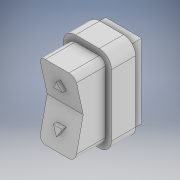
# Autodesk Inventor part: IPC dumb rocker switch
Saved by Autodesk Inventor 2022 (Build 260153000, 153)
## iProperties
Created: 2022-01-05
Part Number: IPC dumb rocker switch
Material: Generic
Document SubType Name: Modeling
Designer: solor
Density: 1 g/cm^3
Appearance: Default
Author: solor
Autodesk Inventor part; units mm, degrees
ref_plane "YZ Plane" through (0, 0, 0) normal (1, 0, 0) x (0, 1, 0)
ref_plane "XZ Plane" through (0, 0, 0) normal (0, 1, 0) x (-1, 0, 0)
ref_plane "XY Plane" through (0, 0, 0) normal (0, 0, 1) x (1, 0, 0)
sketch "Sketch1" plane through (0, 0, 0) normal (0, 0, 1) x (1, 0, 0)
  line L0 (7.88, 0) -> (2, 0)
  arc A0 (7.88, 0) -> (9.88, 2) centre (7.88, 2) ccw
  line L1 (9.88, 17.34) -> (9.88, 2)
  arc A1 (9.88, 17.34) -> (7.88, 19.34) centre (7.88, 17.34) ccw
  line L2 (2, 19.34) -> (7.88, 19.34)
  arc A2 (2, 19.34) -> (0, 17.34) centre (2, 17.34) ccw
  line L3 (0, 2) -> (0, 17.34)
  arc A3 (0, 2) -> (2, 0) centre (2, 2) ccw
  line L4 (0.47, 17.34) -> (0.47, 2)
  arc A4 (0.47, 2) -> (2, 0.47) centre (2, 2) ccw
  line L5 (2, 0.47) -> (7.88, 0.47)
  arc A5 (7.88, 0.47) -> (9.41, 2) centre (7.88, 2) ccw
  line L6 (9.41, 2) -> (9.41, 17.34)
  arc A6 (9.41, 17.34) -> (7.88, 18.87) centre (7.88, 17.34) ccw
  line L7 (7.88, 18.87) -> (2, 18.87)
  arc A7 (2, 18.87) -> (0.47, 17.34) centre (2, 17.34) ccw
  point P0 (0, 0)
  point P1 (0, 0)
  point P2 (0, 0)
  dimension "d0" = 0.47
  constraints: 16 end point, 16 point on circle, 8 centre point, 1 point on line, 7 other
  measures "d0" distance between parallel lines of L3 L4
extrude "Extrusion1" add sketch "Sketch1" along normal blind 13.5 contours A7 L7 A6 L6 A5 L5 A4 L4
sketch "Sketch2" plane through (0, 0, 0) normal (0, 0, -1) x (-1, 0, 0)
  arc A0 (-2, 0.47) -> (-0.47, 2) centre (-2, 2) ccw projected
  line L0 (-0.47, 17.34) -> (-0.47, 2) projected
  arc A1 (-0.47, 17.34) -> (-2, 18.87) centre (-2, 17.34) ccw projected
  line L1 (-7.88, 18.87) -> (-2, 18.87) projected
  arc A2 (-7.88, 18.87) -> (-9.41, 17.34) centre (-7.88, 17.34) ccw projected
  line L2 (-9.41, 2) -> (-9.41, 17.34) projected
  arc A3 (-9.41, 2) -> (-7.88, 0.47) centre (-7.88, 2) ccw projected
  line L3 (-2, 0.47) -> (-7.88, 0.47) projected
  arc A4 (-7.88, 20.37) -> (-10.91, 17.34) centre (-7.88, 17.34) ccw
  line L4 (-7.88, 20.37) -> (-2, 20.37)
  arc A5 (1.03, 17.34) -> (-2, 20.37) centre (-2, 17.34) ccw
  line L5 (1.03, 17.34) -> (1.03, 2)
  arc A6 (-2, -1.03) -> (1.03, 2) centre (-2, 2) ccw
  line L6 (-2, -1.03) -> (-7.88, -1.03)
  arc A7 (-10.91, 2) -> (-7.88, -1.03) centre (-7.88, 2) ccw
  line L7 (-10.91, 2) -> (-10.91, 17.34)
  point P0 (0, 0)
  dimension "d3" = 1.5
  constraints: 8 end point, 8 point on circle, 4 centre point, 7 other
  measures "d3" distance between parallel lines of L2 L7
extrude "Extrusion2" add sketch "Sketch2" against normal blind 6
sketch "Sketch3" plane through (9.41, 2, 13.5) normal (1, 0, 0) x (0, 0, -1)
  line L0 (0, 0) -> (0, 15.34) projected
  line L1 (0, 7.67) -> (2, 7.67) construction
  line L2 (7.5, 16.87) -> (0, 16.87) projected
  line L3 (2, 7.67) -> (0, 16.87)
  line L4 (0, 0) -> (0, -1.53) projected
  line L5 (2, 7.67) -> (0, -1.53)
  line L6 (0, 16.87) -> (0, 15.34) projected
  line L7 (0, 16.87) -> (0, -1.53)
  point P0 (13.5, -2)
  dimension "d6" = 2
  constraints: 8 end point, 1 collinear, 1 horizontal, 1 midpoint
  measures "d6" distance of L1.start L1.end
extrude "Extrusion3" cut sketch "Sketch3" against normal blind 9.175
sketch "Sketch4" plane through (0, 0, 6) normal (0, 0, 1) x (1, 0, 0)
  line L0 (9.41, 9.67) -> (0.47, 9.67) projected
  arc A0 (9.41, 17.34) -> (7.88, 18.87) centre (7.88, 17.34) ccw projected
  line L1 (7.88, 18.87) -> (2, 18.87) projected
  arc A1 (2, 18.87) -> (0.47, 17.34) centre (2, 17.34) ccw projected
  line L2 (0.47, 9.67) -> (0.47, 17.34) projected
  line L3 (9.41, 9.67) -> (0.47, 9.67) projected
  line L4 (9.41, 17.34) -> (9.41, 9.67) projected
  line L5 (13.6871, 9.67) -> (13.6871, 18.87)
  line L6 (4.94, 15.5745) -> (6.0697, 13.6177)
  line L7 (6.0697, 13.6177) -> (3.8103, 13.6177)
  line L8 (3.8103, 13.6177) -> (4.94, 15.5745)
  line L9 (-3.6206, 9.67) -> (18.3642, 9.67)
  line L10 (4.94, 3.7655) -> (6.0697, 5.7223)
  line L11 (6.0697, 5.7223) -> (3.8103, 5.7223)
  line L12 (3.8103, 5.7223) -> (4.94, 3.7655)
  point P0 (0, 0)
  point P1 (4.94, 9.67)
  point P2 (13.6871, 14.27)
  point P3 (4.94, 14.27)
  point P4 (4.94, 14.27)
  point P5 (4.94, 5.07)
  point P6 (4.94, 5.07)
  constraints: 16 end point, 5 symmetric about line, 2 coincident, 2 midpoint, 1 horizontal, 1 vertical, 7 other
extrude "Extrusion4" add sketch "Sketch4" along normal blind 10.7625 contours L6 L7 L8 | L12 L11 L10
sketch "Sketch5" plane through (9.41, 2, 6) normal (1, 0, 0) x (0, 0, -1)
  line L0 (-7.1674, 15.34) -> (-5.5, 7.67) projected
  line L1 (-5.5, 7.67) -> (-7.1674, 0) projected
  line L2 (-8.0469, 15.1488) -> (-6.421, 7.67)
  line L3 (-6.421, 7.67) -> (-8.0469, 0.1912)
  line L4 (-8.0469, 15.1488) -> (-12.9814, 15.34)
  line L5 (-12.9814, 15.34) -> (-12.7678, -1.5252)
  line L6 (-12.7678, -1.5252) -> (-8.0469, 0.1912)
  point P0 (6, -2)
  dimension "d11" = 0.9
  constraints: 10 end point, 1 other
  measures "d11" distance between parallel lines of L0 L2
extrude "Extrusion5" cut sketch "Sketch5" against normal blind 10.7625
sketch "Sketch6" plane through (0, 0, 0) normal (0, 0, -1) x (-1, 0, 0)
  line L0 (1.03, 17.34) -> (1.03, 2) projected
  line L1 (-2, -1.03) -> (-7.88, -1.03) construction
  line L2 (-9.41, 9.67) -> (-0.47, 9.67) construction
  line L3 (-9.88, 19.34) -> (0, 19.34) construction
  line L4 (0, 19.34) -> (0, 0) construction
  line L5 (0, 0) -> (-9.88, 0) construction
  line L6 (-9.88, 0) -> (-9.88, 19.34) construction
  line L7 (-9.88, 19.34) -> (0, 0) construction
  line L8 (0, 19.34) -> (-9.88, 0) construction
  line L9 (-0.47, 18.87) -> (-9.41, 18.87)
  line L10 (-9.41, 18.87) -> (-9.41, 0.47)
  line L11 (-9.41, 0.47) -> (-0.47, 0.47)
  line L12 (-0.47, 0.47) -> (-0.47, 18.87)
  point P0 (1.03, 9.67)
  point P1 (-4.94, -1.03)
  point P2 (-4.94, 9.67)
  dimension "d14" = 9.88
  dimension "d15" = 19.34
  dimension "d16" = 0.47
  constraints: 20 end point, 5 midpoint, 4 parallel, 2 perpendicular, 1 horizontal, 3 other
  measures "d14" distance of L4.end L5.end
  measures "d15" distance of L3.end L4.end
  measures "d16" distance between parallel lines of L3 L9
extrude "Extrusion6" add sketch "Sketch6" along normal blind 3
body "Solid1"
